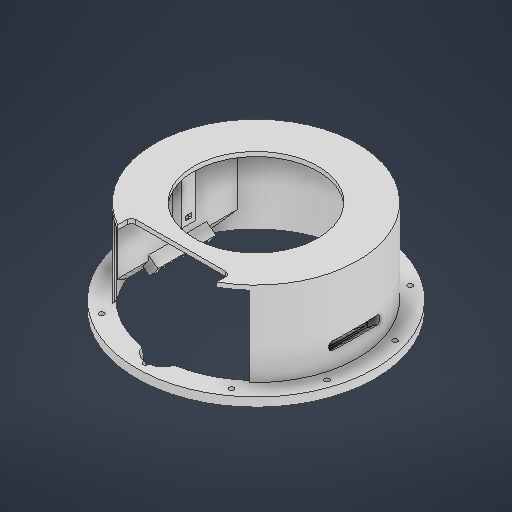
# Autodesk Inventor part: Cylinder Segment  Camera only
Saved by Autodesk Inventor 2025 (Build 290162000, 162)
## iProperties
Created: 2024-04-11
Part Number: Cylinder Segment  Camera only
Material: Generic
Document SubType Name: Modeling
Designer: Thienan Hoang
Density: 1 g/cm^3
Appearance: Default
Author: Thienan Hoang
Autodesk Inventor part; units mm, degrees
ref_plane "YZ Plane" through (0, 0, 0) normal (1, 0, 0) x (0, 1, 0)
ref_plane "XZ Plane" through (0, 0, 0) normal (0, 1, 0) x (-1, 0, 0)
ref_plane "XY Plane" through (0, 0, 0) normal (0, 0, 1) x (1, 0, 0)
sketch "Sketch1" plane through (0, 0, 0) normal (0, 1, 0) x (-1, 0, 0)
  circle A0 centre (0, 0) radius 135
  circle A1 centre (0, 0) radius 115
  circle A2 centre (0, 0) radius 112.0375
  circle A3 centre (0, 0) radius 9.5
  circle A4 centre (0, 0) radius 125
  circle A5 centre (0, -125) radius 2.75
  circle A6 centre (73.4732, -101.1271) radius 2.75
  circle A7 centre (118.8821, -38.6271) radius 2.75
  circle A8 centre (118.8821, 38.6271) radius 2.75
  circle A9 centre (73.4732, 101.1271) radius 2.75
  circle A10 centre (0, 125) radius 2.75
  circle A11 centre (-73.4732, 101.1271) radius 2.75
  circle A12 centre (-118.8821, 38.6271) radius 2.75
  circle A13 centre (-118.8821, -38.6271) radius 2.75
  circle A14 centre (-73.4732, -101.1271) radius 2.75
  dimension "d264" = 250
  dimension "Absolute_Diameter" = 270
  dimension "Diameter_No_Outer_Lip" = 230
  dimension "Inner_Cylinder_Diameter" = 224.075
  dimension "Lip_Diameter" = 19
  dimension "d265" = 5.5
  dimension "d268" = 360
  constraints: 14 centre point, 5 coincident, 1 vertical alignment, 23 other
  measures "Absolute_Diameter" diameter of A0
  measures "Diameter_No_Outer_Lip" diameter of A1
  measures "Inner_Cylinder_Diameter" diameter of A2
  measures "Lip_Diameter" diameter of A3
  measures "d265" diameter of A5
extrude "Extrusion1" add sketch "Sketch1" along normal blind 10 contours A0 | A4 A7 A6 A5 A14 A13 A12 A11 A10 A9 A8
extrude "Extrusion2" add sketch "Sketch1" along normal blind 105.5 contours A1
sketch "Sketch2" plane through (0, 105.5, 0) normal (0, 1, 0) x (1, 0, 0)
  circle A0 centre (0, 0) radius 115
  circle A1 centre (0, 0) radius 70.375
  dimension "Lip_Diameter_Out" = 230
  dimension "Inner_Lip_Diameter" = 140.75
  constraints: 2 centre point, 1 coincident
  measures "Lip_Diameter_Out" diameter of A0
  measures "Inner_Lip_Diameter" diameter of A1
extrude "Extrusion7" add sketch "Sketch2" against normal blind 5
sketch "Sketch28" plane through (0, 10, 0) normal (0, 1, 0) x (1, 0, 0)
  line L0 (-77.5, -75) -> (77.5, -75)
  line L1 (77.5, -75) -> (77.5, -175)
  line L2 (77.5, -175) -> (-77.5, -175)
  line L3 (-77.5, -175) -> (-77.5, -75)
  circle A0 centre (0, -125) radius 2.75 projected
  line L4 (-77.5, -75) -> (77.5, -175) construction
  line L5 (77.5, -75) -> (-77.5, -175) construction
  point P0 (0, 0)
  dimension "d271" = 155
  dimension "d272" = 100
  constraints: 12 end point, 2 midpoint, 2 parallel, 1 horizontal, 1 perpendicular
  measures "d271" distance of L1.end L2.end
  measures "d272" distance of L0.end L1.end
extrude "Extrusion34" cut sketch "Sketch28" along normal up to surface (90.5 mm away)
sketch "Sketch30" plane through (0, 10, 0) normal (0, 1, 0) x (1, 0, 0)
  point P0 (0, 0)
ref_plane "Work Plane19" through (16.25, 10, -160.125) normal (0, 0.3947439, -0.9187912) x (1, 0, 0)
ref_plane "Work Plane21" through (16.25, 10, -160.125) normal (0, 0.911762, 0.4107189) x (1, 0, 0)
ref_plane "Work Plane22" through (16.25, 101.1762, -119.0531) normal (0, 0.911762, 0.4107189) x (1, 0, 0)
sketch "Sketch31" plane through (16.25, 101.1762, -119.0531) normal (0, 0.911762, 0.4107189) x (1, 0, 0)
  circle A0 centre (-16.25, -239.1031) radius 20
  point P0 (-16.25, -150.1031)
  dimension "d286" = 40
  dimension "d289" = 89
  constraints: 1 centre point
  measures "d286" diameter of A0
  measures "d289" distance of point (-16.25, -150.103) A0.centre
extrude "Extrusion36" cut sketch "Sketch31" along normal mid plane 52.8625
fillet "Fillet19" radius 5 2 edges at (-77.5, 55.25, 80.9083) (77.5, 55.25, 80.9083)
sketch "Sketch32" plane through (0, 105.5, 0) normal (0, 1, 0) x (1, 0, 0)
  line L0 (-51, -85) -> (51, -85)
  line L1 (56, -90) -> (56, -125)
  line L2 (56, -125) -> (-56, -125)
  line L3 (-56, -125) -> (-56, -90)
  line L4 (-56, -85) -> (56, -125) construction
  line L5 (56, -85) -> (-56, -125) construction
  arc A0 (-51, -85) -> (-56, -90) centre (-51, -90) ccw
  arc A1 (56, -90) -> (51, -85) centre (51, -90) ccw
  point P0 (0, 0)
  point P1 (0, -105)
  point P2 (0, -85)
  dimension "d291" = 112
  dimension "d292" = 40
  dimension "d293" = 5
  dimension "d294" = 5
  dimension "d295" = 85
  constraints: 12 end point, 4 point on circle, 4 point on line, 4 tangent, 3 midpoint, 2 centre point, 2 parallel, 1 horizontal, 1 perpendicular
  measures "d291" distance of L1.end L2.end
  measures "d292" distance of L5.start L1.end
  measures "d293" radius of A0
  measures "d294" radius of A1
  measures "d295" distance of point (0, 0) point (0, -85)
extrude "Extrusion37" cut sketch "Sketch32" against normal blind 10
sketch "Sketch33" plane through (0, 100.5, 0) normal (0, -1, 0) x (1, 0, 0)
  circle A0 centre (0, 0) radius 70.375
  line L0 (-86.7392, 8) -> (-75, 8)
  line L1 (-75, 8) -> (-75, -8)
  line L2 (-75, -8) -> (-86.7392, -8)
  line L3 (-86.7392, -8) -> (-86.7392, 8)
  line L4 (-86.7392, 8) -> (-75, -8) construction
  line L5 (-75, 8) -> (-86.7392, -8) construction
  line L6 (0, 0) -> (0, 70.375)
  line L7 (86.7392, 8) -> (75, 8)
  line L8 (75, 8) -> (75, -8)
  line L9 (75, -8) -> (86.7392, -8)
  line L10 (86.7392, -8) -> (86.7392, 8)
  line L11 (86.7392, 8) -> (75, -8) construction
  line L12 (75, 8) -> (86.7392, -8) construction
  circle A1 centre (0, 0) radius 76.375
  point P0 (-80.8696, 0)
  point P1 (80.8696, 0)
  point P2 (-75, 0)
  point P3 (-75.9549, -8)
  point P4 (-75.9549, 8)
  point P5 (75.9549, 8)
  point P6 (75.9549, -8)
  dimension "d313" = 140.75
  dimension "d298" = 16
  dimension "d301" = 75
  dimension "d314" = 6
  constraints: 26 end point, 5 symmetric about line, 3 midpoint, 2 parallel, 1 centre point, 1 coincident, 1 horizontal, 1 perpendicular, 1 vertical, 1 vertical alignment, 2 other
  measures "d298" distance of L0.end L1.end
  measures "d301" distance of point (0, 0) point (-75, 0)
extrude "Extrusion38" add sketch "Sketch33" along normal blind 45 contours L0 A1 L2 L3 | L7 L10 L9 A1
sketch "Sketch35" plane through (0, 55.5, 0) normal (0, -1, 0) x (1, 0, 0)
  line L0 (0, 0) -> (0, 42.8625)
  arc A0 (80.604, -8) -> (-80.604, -8) centre (0, 0) ccw
  circle A1 centre (-81, 0) radius 3.5625
  circle A2 centre (81, 0) radius 3.5625
  line L1 (-82.978, -3.6069) -> (-85.1126, -0.0905)
  line L2 (-85.1126, -0.0905) -> (-83.1347, 3.5164)
  line L3 (-83.1347, 3.5164) -> (-79.022, 3.6069)
  line L4 (-79.022, 3.6069) -> (-76.8874, 0.0905)
  line L5 (-76.8874, 0.0905) -> (-78.8653, -3.5164)
  line L6 (-78.8653, -3.5164) -> (-82.978, -3.6069)
  line L7 (82.978, -3.6069) -> (85.1126, -0.0905)
  line L8 (85.1126, -0.0905) -> (83.1347, 3.5164)
  line L9 (83.1347, 3.5164) -> (79.022, 3.6069)
  line L10 (79.022, 3.6069) -> (76.8874, 0.0905)
  line L11 (76.8874, 0.0905) -> (78.8653, -3.5164)
  line L12 (78.8653, -3.5164) -> (82.978, -3.6069)
  arc A3 (75.9549, -8) -> (-75.9549, -8) centre (0, 0) ccw
  line L13 (-75.9549, -8) -> (-86.7392, -8)
  line L14 (-86.7392, -8) -> (-86.7392, 8)
  line L15 (86.7392, -8) -> (86.7392, 8)
  line L16 (-86.7392, 8) -> (-75.9549, 8) projected
  line L17 (-86.7392, 8) -> (-75.9549, 8)
  line L18 (86.7392, 8) -> (75.9549, 8)
  line L19 (-79.022, 3.6069) -> (-78.8653, -3.5164)
  line L20 (-78.8653, -3.5164) -> (-14.3502, -2.0973)
  line L21 (-14.3502, -2.0973) -> (-14.5068, 5.0259)
  line L22 (-14.5068, 5.0259) -> (-79.022, 3.6069)
  line L23 (79.022, 3.6069) -> (78.8653, -3.5164)
  line L24 (78.8653, -3.5164) -> (65.0181, -3.2118)
  line L25 (65.0181, -3.2118) -> (65.1748, 3.9115)
  line L26 (65.1748, 3.9115) -> (79.022, 3.6069)
  line L27 (86.7392, -8) -> (75.9549, -8)
  arc A4 (87.1335, -8) -> (-87.1335, -8) centre (0, 0) ccw
  point P0 (-80.9217, -3.5616)
  point P1 (-76.2966, -3.4599)
  point P2 (-76.2869, 3.667)
  point P3 (76.2869, 3.667)
  point P4 (76.2966, -3.4599)
  dimension "d309" = 7.125
  dimension "d308" = 162
  constraints: 54 end point, 10 symmetric about line, 8 point on circle, 5 equal length, 4 centre point, 4 coincident, 4 point on line, 3 perpendicular, 1 horizontal, 1 midpoint, 1 vertical, 17 other
  measures "d308" diameter of A0
extrude "Extrusion40" cut sketch "Sketch35" against normal blind 15 contours A2 L23 A0 | A0 A2 | A2 L23 | A1 L19 A0 | A0 A1 | A1 L19
extrude "Extrusion41" add sketch "Sketch35" along normal blind 5 contours L27 A3 L24 L12 A0 | A0 L12 L7 L8 L9 A2 L18 L15 L27 | L9 L26 A3 L18 A0 | L16 A3 L22 L3 A0 | A0 A1 L3 L2 L1 L6 L13 L14 L16 | L6 L20 A3 L13 A0
sketch "Sketch36" plane through (0, 50.5, 0) normal (0, -1, 0) x (1, 0, 0)
  circle A0 centre (0, 0) radius 76.375
  line L0 (-86.7392, 8) -> (-75.9549, 8) projected
  line L1 (-86.7392, -8) -> (-86.7392, 8) projected
  line L2 (-86.7392, 8) -> (-86.7392, -8)
  line L3 (-86.7392, -8) -> (-75.9549, -8)
  line L4 (-75.9549, 8) -> (-86.7392, 8)
  arc A1 (-80.9217, -3.5616) -> (-81.0783, 3.5616) centre (-81, 0) ccw projected
  circle A2 centre (-81, 0) radius 3.5667
  line L5 (0, 0) -> (0, 76.375)
  line L6 (86.7392, 8) -> (75.9549, 8)
  line L7 (86.7392, -8) -> (86.7392, 8)
  line L8 (86.7392, 8) -> (86.7392, -8)
  line L9 (86.7392, -8) -> (75.9549, -8)
  line L10 (75.9549, 8) -> (86.7392, 8)
  arc A3 (81.0783, 3.5616) -> (80.9217, -3.5616) centre (81, 0) ccw
  circle A4 centre (81, 0) radius 3.5667
  constraints: 18 end point, 9 symmetric about line, 4 centre point, 3 coincident, 3 point on circle, 2 equal length, 1 perpendicular, 1 vertical, 2 other
extrude "Extrusion42" add sketch "Sketch36" along normal blind 5 contours A0 L6 L7 L9 | L3 L1 L0 A0
sketch "Sketch37" plane through (0, 0, 0) normal (0, -1, 0) x (1, 0, 0)
  arc A0 (-15.9123, 110.9018) -> (15.9123, 110.9018) centre (0, 0) ccw projected
  line L0 (-135.2345, 68.2625) -> (-88.8405, 68.2625)
  line L1 (-88.8405, 68.2625) -> (-88.8405, -68.2625)
  line L2 (-88.8405, -68.2625) -> (-135.2345, -68.2625)
  line L3 (-135.2345, -68.2625) -> (-135.2345, 68.2625)
  line L4 (-135.2345, 68.2625) -> (-88.8405, -68.2625) construction
  line L5 (-88.8405, 68.2625) -> (-135.2345, -68.2625) construction
  circle A1 centre (0, 0) radius 135 projected
  line L6 (0, 135) -> (0, -135)
  line L7 (135.2345, 68.2625) -> (88.8405, 68.2625)
  line L8 (88.8405, 68.2625) -> (88.8405, -68.2625)
  line L9 (88.8405, -68.2625) -> (135.2345, -68.2625)
  line L10 (135.2345, -68.2625) -> (135.2345, 68.2625)
  line L11 (-112.0375, 0) -> (-112.0375, -68.2625)
  line L12 (-112.0375, 0) -> (-112.0375, 68.2625)
  line L13 (112.0375, 0) -> (112.0375, -68.2625)
  line L14 (112.0375, 0) -> (112.0375, 68.2625)
  constraints: 30 end point, 7 symmetric about line, 4 midpoint, 4 point on circle, 2 parallel, 1 horizontal, 1 perpendicular, 1 vertical
extrude "Extrusion43" add sketch "Sketch37" against normal up to surface (100.5 mm away) contours L1 A0 | L8 A0
chamfer "Chamfer14" distance 15 distance2 20 2 edges at (-88.8405, 0, 0) (88.8405, 0, 0) measured on face at (-89.3405, 0, 0) measured on face at (89.3405, 0, 0)
sketch "Sketch38" plane through (-88.8405, 20, 68.2625) normal (0.8, -0.6, 0) x (0, 0, -1)
  line L0 (136.525, 0) -> (0, 0) projected
  line L1 (68.2625, 0) -> (68.2625, -25)
  line L2 (26.1964, -25) -> (110.3286, -25) projected
  line L3 (42.8625, 32.0789) -> (42.8625, -38.0789)
  arc A0 (42.8625, -0.75) -> (42.8625, -5.25) centre (42.8625, -3) ccw
  arc A1 (93.6625, -5.25) -> (93.6625, -0.75) centre (93.6625, -3) ccw
  line L4 (42.8625, -7) -> (68.2625, -7)
  line L5 (42.8625, -5.25) -> (68.2625, -5.25)
  line L6 (42.8625, -0.75) -> (68.2625, -0.75)
  line L7 (42.8625, 1) -> (68.2625, 1)
  line L8 (93.6625, -7) -> (68.2625, -7)
  line L9 (93.6625, -5.25) -> (68.2625, -5.25)
  line L10 (93.6625, -0.75) -> (68.2625, -0.75)
  line L11 (93.6625, 1) -> (68.2625, 1)
  arc A2 (93.6625, -7) -> (93.6625, 1) centre (93.6625, -3) ccw
  arc A3 (91.0167, 0) -> (90.3553, -0.75) centre (93.6625, -3) ccw
  arc A4 (46.1697, -0.75) -> (45.5083, 0) centre (42.8625, -3) ccw
  arc A5 (42.8625, 1) -> (42.8625, -7) centre (42.8625, -3) ccw
  point P0 (68.2625, 37.3043)
  dimension "d324" = 25.4
  dimension "d330" = 4.5
  dimension "d341" = 22
  dimension "d361" = 1.75
  constraints: 20 end point, 12 point on circle, 11 point on line, 6 centre point, 6 symmetric about line, 4 tangent, 3 midpoint, 3 parallel, 2 coincident, 2 perpendicular, 1 other
  measures "d324" distance between parallel lines of L1 L3
  measures "d330" diameter of A0
  measures "d341" distance from line of L2 A4.centre
  measures "d361" distance between parallel lines of L6 L7
extrude "Extrusion44" cut sketch "Sketch38" against normal through all contours A3 L10 L1 L0 | L0 L3 L7 L11 A2 | L0 A2 L8 L1 L9 A1 L10 A3 | L1 L6 A4 L0 | L10 A1 L9 L1 | A4 L6 L3 L0 | L1 L5 L3 L6 | L3 A0 A5 L0 | L0 A5 L3 | L1 L4 L3 L5 | L3 A0
extrude "Extrusion45" add sketch "Sketch38" against normal blind 8 contours A3 L10 L1 L0 | L0 L3 L7 L11 A2 | L0 A2 L8 L1 L9 A1 L10 A3 | L1 L6 A4 L0 | A4 L6 L3 L0 | L3 A0 A5 L0 | L0 A5 L3 | L1 L4 L3 L5
sketch "Sketch39" plane through (88.8405, 20, -68.2625) normal (-0.8, -0.6, 0) x (0, 0, 1)
  line L0 (136.525, 0) -> (0, 0) projected
  line L1 (68.2625, 0) -> (68.2625, -25)
  line L2 (26.1964, -25) -> (110.3286, -25) projected
  line L3 (42.8625, 32.0789) -> (42.8625, -38.0789)
  circle A0 centre (42.8625, -3) radius 3.75
  circle A1 centre (42.8625, -3) radius 2.25
  circle A2 centre (93.6625, -3) radius 3.75
  circle A3 centre (93.6625, -3) radius 2.25
  line L4 (68.2625, 0) -> (68.2625, 14.9827)
  line L5 (42.8625, 0.75) -> (68.2625, 0.75)
  line L6 (42.8625, 0.75) -> (68.2625, 0.75) construction
  line L7 (42.8625, -6.75) -> (68.2625, -6.75)
  line L8 (93.6625, 0.75) -> (68.2625, 0.75)
  line L9 (93.6625, -6.75) -> (68.2625, -6.75)
  line L10 (42.8625, -5.25) -> (93.6625, -5.25)
  line L11 (42.8625, -0.75) -> (93.6625, -0.75)
  point P0 (68.2625, 37.3043)
  point P1 (93.6625, -6.75)
  point P2 (93.6625, 0.75)
  dimension "d333" = 25.4
  dimension "d334" = 7.5
  dimension "d335" = 4.5
  dimension "d340" = 22
  dimension "d360" = 0
  constraints: 20 end point, 6 point on circle, 4 centre point, 4 point on line, 4 symmetric about line, 3 midpoint, 3 tangent, 2 coincident, 2 parallel, 2 perpendicular, 1 collinear, 1 horizontal, 1 vertical, 2 other
  measures "d333" distance between parallel lines of L1 L3
  measures "d334" diameter of A0
  measures "d335" diameter of A1
  measures "d340" distance from line of L2 A0.centre
  measures "d360" distance between parallel lines of L5 L6
extrude "Extrusion46" cut sketch "Sketch39" against normal through all contours A2 L10 A3 L11 L0 | L0 A2 | A2 L11 L1 L0 | L0 L4 L8 A2 | L1 L11 A0 L0 | L0 A0 L5 L4 | L11 A3 L10 A2 | A2 L10 L1 L11 | L9 L1 L10 A2 | A0 L11 L3 L0 | L0 L3 A0 | L1 L10 A0 L11 | A3 | L7 A0 L10 L1 | L3 L0 A0 | L3 A1 A0 L0 | A0 L10 A1 L11 | L3 L10 A0 | A1 L3 | L3 A1
extrude "Extrusion47" add sketch "Sketch39" against normal blind 8 contours A2 L10 A3 L11 L0 | L0 A2 | A2 L11 L1 L0 | L0 L4 L8 A2 | L1 L11 A0 L0 | L0 A0 L5 L4 | L9 L1 L10 A2 | A0 L11 L3 L0 | L0 L3 A0 | L7 A0 L10 L1 | L3 L0 A0 | L3 A1 A0 L0 | L3 L10 A0
sketch "Sketch43" plane through (103.8405, 0, -42.0661) normal (-0.8, -0.6, 0) x (0, 0, 1)
  line L0 (9.1661, 14.5) -> (24.1661, 14.5)
  line L1 (24.1661, 29.5) -> (9.1661, 29.5)
  line L2 (9.1661, 29.5) -> (9.1661, 14.5)
  arc A0 (16.6661, 24.25) -> (16.6661, 19.75) centre (16.6661, 22) ccw projected
  line L3 (9.1661, 14.5) -> (24.1661, 29.5) construction
  line L4 (24.1661, 14.5) -> (9.1661, 29.5) construction
  line L5 (59.9661, 14.5) -> (74.9661, 14.5)
  line L6 (74.9661, 14.5) -> (74.9661, 29.5)
  line L7 (74.9661, 29.5) -> (59.9661, 29.5)
  line L8 (59.9661, 14.5) -> (74.9661, 29.5) construction
  line L9 (74.9661, 14.5) -> (59.9661, 29.5) construction
  circle A1 centre (67.4661, 22) radius 2.25
  line L10 (24.1661, 29.5) -> (59.9661, 29.5)
  line L11 (24.1661, 14.5) -> (59.9661, 14.5)
  line L12 (16.6661, 24.25) -> (67.4661, 24.25)
  line L13 (16.6661, 19.75) -> (67.4661, 19.75) projected
  line L14 (16.6661, 19.75) -> (67.4661, 19.75)
  point P0 (42.0661, 62.3043)
  dimension "d352" = 15
  dimension "d353" = 15
  dimension "d354" = 15
  dimension "d355" = 15
  constraints: 28 end point, 4 midpoint, 3 parallel, 2 collinear, 2 horizontal, 2 tangent, 1 centre point, 1 coincident, 1 perpendicular, 1 point on circle
  measures "d352" distance of L1.end L1.start
  measures "d353" distance of L1.start L0.end
  measures "d354" distance of L7.end L6.end
  measures "d355" distance of L6.end L5.end
sketch "Sketch42" plane through (-88.8405, 20, 68.2625) normal (0.8, -0.6, 0) x (0, 0, -1)
  arc A0 (42.8625, -0.75) -> (42.8625, -5.25) centre (42.8625, -3) ccw projected
  circle A1 centre (42.8625, -3) radius 2.25
  arc A2 (93.6625, -5.25) -> (93.6625, -0.75) centre (93.6625, -3) ccw projected
  circle A3 centre (93.6625, -3) radius 2.25
  line L0 (35.3625, 4.5) -> (35.3625, -10.5)
  line L1 (35.3625, -10.5) -> (50.3625, -10.5)
  line L2 (50.3625, 4.5) -> (35.3625, 4.5)
  line L3 (35.3625, 4.5) -> (50.3625, -10.5) construction
  line L4 (35.3625, -10.5) -> (50.3625, 4.5) construction
  line L5 (101.1625, 4.5) -> (86.1625, 4.5)
  line L6 (86.1625, -10.5) -> (101.1625, -10.5)
  line L7 (101.1625, -10.5) -> (101.1625, 4.5)
  arc A4 (93.6625, -7) -> (93.6625, 1) centre (93.6625, -3) ccw projected
  line L8 (101.1625, 4.5) -> (86.1625, -10.5) construction
  line L9 (86.1625, 4.5) -> (101.1625, -10.5) construction
  line L10 (50.3625, 4.5) -> (86.1625, 4.5)
  line L11 (50.3625, -10.5) -> (86.1625, -10.5)
  line L12 (42.8625, -0.75) -> (93.6625, -0.75)
  line L13 (93.6625, -5.25) -> (42.8625, -5.25)
  point P0 (68.2625, 37.3043)
  dimension "d344" = 15
  dimension "d345" = 15
  dimension "d346" = 15
  dimension "d347" = 15
  constraints: 28 end point, 5 parallel, 5 tangent, 4 midpoint, 2 centre point, 2 coincident, 1 collinear, 1 horizontal, 1 perpendicular, 1 vertical
  measures "d344" distance of L0.start L0.end
  measures "d345" distance of L1.end L0.end
  measures "d346" distance of L5.start L5.end
  measures "d347" distance of L6.start L5.end
extrude "Extrusion49" add sketch "Sketch42" along normal blind 10 and the other way blind 5
extrude "Extrusion50" add sketch "Sketch43" along normal blind 10 and the other way blind 5
body "Solid1"
